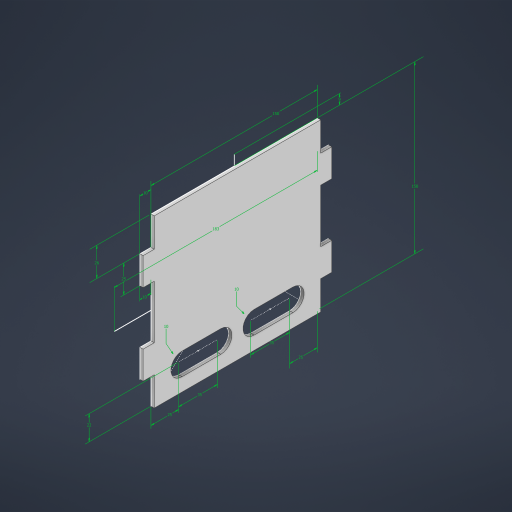
# Autodesk Inventor part: back_part
Saved by Autodesk Inventor 2023 (Build 270158000, 158)
## iProperties
Created: 2022-11-27
Part Number: back_part
Material: Generic
Document SubType Name: Modeling
Designer: washington
Density: 1 g/cm^3
Appearance: Default
Author: washington
Autodesk Inventor part; units mm, degrees
ref_plane "YZ Plane" through (0, 0, 0) normal (1, 0, 0) x (0, 1, 0)
ref_plane "XZ Plane" through (0, 0, 0) normal (0, 1, 0) x (-1, 0, 0)
ref_plane "XY Plane" through (0, 0, 0) normal (0, 0, 1) x (1, 0, 0)
sketch "Sketch1" plane through (0, 0, 0) normal (1, 0, 0) x (0, 1, 0)
  line L0 (75, 75) -> (75, -75)
  line L1 (-75, -75) -> (-75, 75)
  line L2 (-75, 75) -> (75, -75) construction
  line L3 (75, 75) -> (-75, -75) construction
  line L4 (-53, 50) -> (-53, 15) construction
  line L5 (-63, 50) -> (-63, 15)
  line L6 (-43, 15) -> (-43, 50)
  arc A0 (-43, 50) -> (-63, 50) centre (-53, 50) ccw
  arc A1 (-63, 15) -> (-43, 15) centre (-53, 15) ccw
  line L7 (-53, -15) -> (-53, -50) construction
  line L8 (-43, -15) -> (-43, -50)
  line L9 (-63, -50) -> (-63, -15)
  arc A2 (-43, -15) -> (-63, -15) centre (-53, -15) ccw
  arc A3 (-63, -50) -> (-43, -50) centre (-53, -50) ccw
  line L10 (49, 75) -> (49, 85)
  line L11 (49, 85) -> (24, 85)
  line L12 (24, 85) -> (24, 75)
  line L13 (0, 0) -> (0, 108)
  line L14 (-49, 75) -> (-49, 85)
  line L15 (-49, 85) -> (-24, 85)
  line L16 (-24, 85) -> (-24, 75)
  line L17 (0, 0) -> (84, 0)
  line L18 (49, -75) -> (49, -85)
  line L19 (49, -85) -> (24, -85)
  line L20 (24, -85) -> (24, -75)
  line L21 (-49, -75) -> (-49, -85)
  line L22 (-49, -85) -> (-24, -85)
  line L23 (-24, -85) -> (-24, -75)
  line L24 (49, 75) -> (75, 75)
  line L25 (-75, 75) -> (-49, 75)
  line L26 (-24, 75) -> (24, 75)
  line L27 (75, -75) -> (49, -75)
  line L28 (24, -75) -> (-24, -75)
  line L29 (-49, -75) -> (-75, -75)
  point P0 (-53, 32.5)
  point P1 (-53, -32.5)
  dimension "d0" = 150
  dimension "d1" = 150
  dimension "d2" = 25
  dimension "d4" = 25
  dimension "d5" = 35
  dimension "d6" = 35
  dimension "d7" = 22
  dimension "d8" = 10
  dimension "d9" = 10
  dimension "d12" = 25
  dimension "d13" = 26
  dimension "d14" = 10
  dimension "d15" = 10
  dimension "d16" = 9
  dimension "d17" = 183
  constraints: 64 end point, 12 parallel, 12 symmetric about line, 8 point on circle, 8 tangent, 7 perpendicular, 4 centre point, 4 horizontal, 4 midpoint, 3 vertical, 2 point on line
  measures "d0" distance of L0.start L0.end
  measures "d1" distance of L0.end L1.start
  measures "d2" vertical distance of L4.start L1.end
  measures "d4" vertical distance of L7.end L1.start
  measures "d5" distance of L4.end L4.start
  measures "d6" distance of L7.end L7.start
  measures "d7" horizontal distance of L4.start L1.end
  measures "d8" radius of A0
  measures "d9" radius of A2
  measures "d12" distance of L10.end L11.end
  measures "d13" distance between parallel lines of L10 L0
  measures "d14" distance of L12.end L11.end
  measures "d15" distance between parallel lines of L11 L24
  measures "d16" distance from line of L17.end L0
  measures "d17" distance from line of L13.end L27
extrude "Extrusion1" add sketch "Sketch1" along normal blind 3
body "Solid1"
